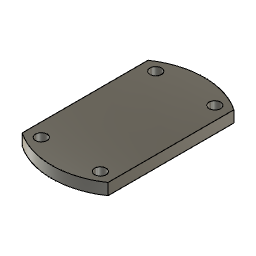
_Selfy Stick head.aeb56935-b141-4065-bd1e-c25a75e71f95_LV0 (Autodesk Fusion 360 design; units mm, degrees)
Autodesk Fusion 360 part; units mm, degrees
sketch "Sketch1" plane through (0, 0, 0) normal (0, 0, 1) x (1, 0, 0) in component "Base"
  circle A0 centre (0, 0) radius 12
  dimension "d33" = 24
  constraint coincident A0.centre origin
  measures "d33" diameter of A0
extrude "Extrude1" add sketch "Sketch1" along normal blind 41 makes body 1 in component "Base"
ref_plane "WorkPlane1" through (0, -12, 17.2236) normal (0, -1, 0) x (-1, 0, 0) in component "Base"
sketch "Sketch2" plane through (0, -12, 17.2236) normal (0, -1, 0) x (1, 0, 0) in component "Base"
  line L0 (12, -17.2236) -> (-12, -17.2236)
  line L1 (12, 23.7764) -> (-12, 23.7764)
  line L2 (-17.778, -9.2236) -> (25, -9.2236) construction
  line L3 (-17.5615, 10.2764) -> (25, 10.2764) construction
  circle A0 centre (-0.0008, -6.7236) radius 2.5
  circle A1 centre (-0.0008, -6.7236) radius 1.5
  circle A2 centre (-0.0002, 13.7764) radius 3.5
  dimension "d37" = 24
  dimension "d38" = 41
  dimension "d39" = 8
  dimension "d40" = 27.5
  dimension "d42" = 5
  dimension "d43" = 10.5
  dimension "d44" = 3
  dimension "d45" = 7
  dimension "d46" = 31
  constraint horizontal L2
  constraint horizontal L3
  constraint concentric A0 A1
  measures "d37" distance of L0.start L0.end
  measures "d38" distance of L0 L1
  measures "d39" distance of L0 L2
  measures "d40" distance of L0 L3
  measures "d42" diameter of A0
  measures "d43" distance of L0 A0.centre
  measures "d44" diameter of A1
  measures "d45" diameter of A2
  measures "d46" distance of L0 A2.centre
extrude "Extrude2" cut sketch "Sketch2" against normal blind 24 contours A1 | A2 bodies 1 in component "Base"
ref_plane "WorkPlane2" through (0, -12, 12.6145) normal (0, -1, 0) x (-1, 0, 0) in component "Base"
sketch "Sketch3" plane through (0, -12, 12.6145) normal (0, -1, 0) x (1, 0, 0) in component "Base"
  line L0 (12, -12.6145) -> (-12, -12.6145)
  circle A0 centre (0, -2.1) radius 2.5
  dimension "d51" = 5
  measures "d51" diameter of A0
extrude "Extrude3" cut sketch "Sketch3" against normal blind 3 bodies 1 in component "Base"
fillet "Fillet1" radius 10 1 edges at (-11.1879, -4.3394, 41) on bodies 1 in component "Base"
ref_plane "WorkPlane6" through (0, 0, 41) normal (0, 0, 1) x (1, 0, 0) in component "Base"
sketch "Sketch4" plane through (0, 0, 41) normal (0, 0, 1) x (1, 0, 0) in component "Base"
  line L0 (-14, 4.5) -> (14, 4.5)
  line L1 (14, 4.5) -> (14, -4.5)
  line L2 (14, -4.5) -> (-14, -4.5)
  line L3 (-14, -4.5) -> (-14, 4.5)
  line L4 (-14, 4.5) -> (14, -4.5) construction
  line L5 (14, 4.5) -> (-14, -4.5) construction
  dimension "d60" = 9
  constraint horizontal L0
  constraint perpendicular L0 L1
  constraint parallel L0 L2
  constraint parallel L1 L3
  constraint coincident L4 origin
  constraint coincident L5 origin
  measures "d60" distance of L0.end L1.end
extrude "Extrude4" cut sketch "Sketch4" against normal blind 22 bodies 1 in component "Base"
ref_plane "WorkPlane7" through (0, 12, 20.5561) normal (0, 1, 0) x (1, 0, 0) in component "Base"
sketch "Sketch5" plane through (0, 12, 20.5561) normal (0, 1, 0) x (1, 0, 0) in component "Base"
  line L0 (-3.628, -12.9566) -> (0.3454, -14.8465)
  line L1 (0.3454, -14.8465) -> (3.9689, -12.3504)
  line L2 (3.9689, -12.3504) -> (3.6189, -7.9643)
  line L3 (3.6189, -7.9643) -> (-0.3546, -6.0744)
  line L4 (-0.3546, -6.0744) -> (-3.978, -8.5706)
  line L5 (-3.978, -8.5706) -> (-3.628, -12.9566)
  point P0 (-0.0046, -10.4605)
  dimension "d64" = 4.4
  measures "d64" distance of L0.start P0
extrude "Extrude5" cut sketch "Sketch5" against normal up to surface (7.5 mm away) bodies 1 in component "Base"
ref_plane "WorkPlane8" through (0, 12, 4.5743) normal (0, 1, 0) x (1, 0, 0) in component "Base"
sketch "Sketch6" plane through (0, 12, 4.5743) normal (0, 1, 0) x (1, 0, 0) in component "Base"
  circle A0 centre (-0.0008, -5.9257) radius 1.5
  line L0 (-2.8139, -4.6232) -> (-2.5353, -7.7106)
  line L1 (-2.5353, -7.7106) -> (0.2778, -9.0131)
  line L2 (0.2778, -9.0131) -> (2.8123, -7.2282)
  line L3 (2.8123, -7.2282) -> (2.5338, -4.1407)
  line L4 (2.5338, -4.1407) -> (-0.2793, -2.8382)
  line L5 (-0.2793, -2.8382) -> (-2.8139, -4.6232)
  point P0 (-0.0008, -5.9257)
  dimension "d68" = 3
  dimension "d69" = 3.1
  constraint coincident P0 A0.centre
  measures "d68" diameter of A0
  measures "d69" distance of L0.start P0
extrude "Extrude6" cut sketch "Sketch6" against normal blind 2.6 bodies 1 in component "Base"
ref_plane "WorkPlane10" through (0, 0, 0) normal (0, 0, -1) x (-1, 0, 0) in component "Base"
sketch "Sketch7" plane through (0, 0, 0) normal (0, 0, -1) x (1, 0, 0) in component "Base"
  circle A0 centre (0, 0) radius 6.5
  dimension "d74" = 13
  constraint coincident A0.centre origin
  measures "d74" diameter of A0
extrude "Extrude7" cut sketch "Sketch7" against normal blind 18 bodies 1 in component "Base"
sketch "Sketch1 (2)" plane through (0, 0, 0) normal (0, 0, 1) x (1, 0, 0) in component "Top bottom half"
  line L0 (22.2214, 3.672) -> (22.2214, 36.672)
  line L1 (-0.2786, 36.672) -> (-0.2786, 3.672)
  line L2 (-0.2786, 36.672) -> (22.2214, 36.672) construction
  line L3 (-0.2786, 3.672) -> (22.2214, 3.672) construction
  line L4 (10.9714, 40.172) -> (10.9714, 0.172) construction
  arc A0 (22.2214, 36.672) -> (-0.2786, 36.672) centre (10.9714, 20.1725) ccw
  arc A1 (-0.2786, 3.672) -> (22.2214, 3.672) centre (10.9714, 20.0024) ccw
  line L5 (4.7214, 36.672) -> (4.7214, 3.672) construction
  line L6 (17.2214, 36.672) -> (17.2214, 3.672) construction
  circle A2 centre (3.2214, 35.172) radius 1.5
  circle A3 centre (18.7214, 35.172) radius 1.5
  circle A4 centre (3.2214, 5.172) radius 1.5
  circle A5 centre (18.7214, 5.172) radius 1.5
  dimension "d82" = 22.5
  dimension "d83" = 40
  dimension "d84" = 6.25
  dimension "d85" = 11.25
  dimension "d86" = 6.25
  dimension "d88" = 3.5
  dimension "d89" = 3.5
  dimension "d90" = 3
  dimension "d91" = 1.5
  dimension "d92" = 1.5
  dimension "d93" = 3
  dimension "d94" = 1.5
  dimension "d95" = 1.5
  dimension "d96" = 3
  dimension "d97" = 1.5
  dimension "d98" = 1.5
  dimension "d99" = 3
  dimension "d100" = 1.5
  dimension "d101" = 1.5
  constraint vertical L0
  constraint vertical L1
  constraint perpendicular L0 L2
  constraint perpendicular L0 L3
  constraint coincident L4.end A1
  constraint coincident L2 L5.start
  constraint coincident L3 L5.end
  constraint perpendicular L3 L5
  constraint coincident L2 L6.start
  constraint coincident L3 L6.end
  constraint perpendicular L3 L6
  measures "d82" distance of L1.start L0.end
  measures "d83" distance of L4.start L4.end
  measures "d84" distance of L4 L5
  measures "d85" distance of L1 L4
  measures "d86" distance of L4 L6
  measures "d88" distance of L3 L4.end
  measures "d89" distance of L2 L4.start
  measures "d90" diameter of A2
  measures "d91" distance of L2 A2.centre
  measures "d92" distance of L5 A2.centre
  measures "d93" diameter of A3
  measures "d94" distance of L2 A3.centre
  measures "d95" distance of L6 A3.centre
  measures "d96" diameter of A4
  measures "d97" distance of L3 A4.centre
  measures "d98" distance of L5 A4.centre
  measures "d99" diameter of A5
  measures "d100" distance of L6 A5.centre
  measures "d101" distance of L3 A5.centre
extrude "Extrude1'" add sketch "Sketch1 (2)" along normal blind 3 separate body makes body 2 in component "Top bottom half"
component "Top bottom half" placed x (1, 0, 0) y (0, 1, 0) z (0, 0, 1) at (0, 0, 0)
component "Base" placed x (1, 0, 0) y (0, 1, 0) z (0, 0, 1) at (0, 0, 0)
